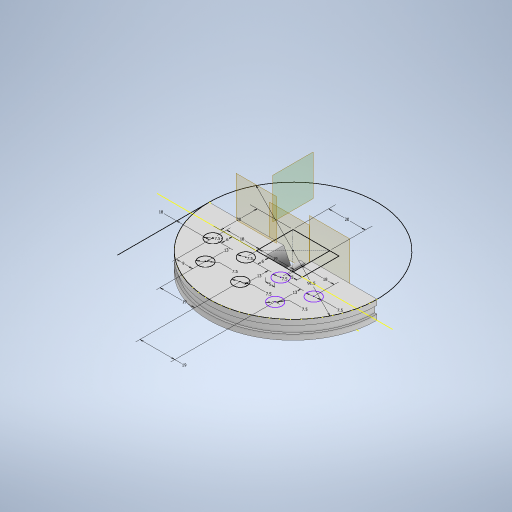
# Autodesk Inventor part: new탄두윗판구멍1_2
Saved by Autodesk Inventor 2023 (Build 270158000, 158)
## iProperties
Created: 2023-10-30
Part Number: new탄두윗판구멍1_2
Material: 일반
Document SubType Name: Modeling
Designer: rlatk
Density: 1 g/cm^3
Appearance: 기본값
Author: rlatk
Autodesk Inventor part; units mm, degrees
ref_plane "YZ Plane" through (0, 0, 0) normal (1, 0, 0) x (0, 1, 0)
ref_plane "XZ Plane" through (0, 0, 0) normal (0, 1, 0) x (-1, 0, 0)
ref_plane "XY Plane" through (0, 0, 0) normal (0, 0, 1) x (1, 0, 0)
sketch "스케치1" plane through (0, 0, 0) normal (0, 1, 0) x (-1, 0, 0)
  line L0 (-10, 10) -> (10, 10)
  line L1 (10, 10) -> (10, -10)
  line L2 (10, -10) -> (-10, -10)
  line L3 (-10, -10) -> (-10, 10)
  line L4 (-10, 10) -> (10, -10) construction
  line L5 (10, 10) -> (-10, -10) construction
  line L6 (-10, -10) -> (-15, -10)
  line L7 (-15, -10) -> (-15, 10)
  line L8 (-15, 10) -> (-10, 10)
  line L9 (-10, 10) -> (-10, -10)
  circle A0 centre (0, 0) radius 45.75
  dimension "d0" = 20
  dimension "d1" = 20
  dimension "d2" = 5
  dimension "d17" = 91.5
  constraints: 20 end point, 4 parallel, 2 horizontal, 2 midpoint, 2 perpendicular, 1 centre point, 1 coincident
  measures "d0" distance of L1.end L2.end
  measures "d1" distance of L0.end L1.end
  measures "d2" distance of L7.end L8.end
  measures "d17" diameter of A0
ref_plane "작업 평면2" through (-10, 20, -10) normal (-1, 0, 0) x (0, 0, 1)
sketch "스케치2" plane through (-10, 20, -10) normal (-1, 0, 0) x (0, 0, 1)
  line L0 (20, -100) -> (20, 0) projected
  line L1 (0, 0) -> (20, 0) projected
  line L2 (0, 0) -> (0, -100) projected
  line L3 (20, -100) -> (0, -100) projected
  circle A0 centre (10, -91) radius 4.5
  point P0 (10, -20)
  dimension "d7" = 9
  dimension "d8" = 9
  constraints: 1 centre point
  measures "d7" diameter of A0
  measures "d8" distance from line of L3 A0.centre
ref_plane "작업 평면1" through (-10, 20, 10) normal (0, 0, 1) x (1, 0, 0)
sketch "스케치3" plane through (-10, 20, 10) normal (0, 0, 1) x (1, 0, 0)
  line L0 (20, -20) -> (25, -20) projected
  line L1 (25, -20) -> (25, 0) projected
  line L2 (0, 0) -> (25, 0) projected
  line L3 (0, -100) -> (0, 0) projected
  line L4 (20, -100) -> (0, -100) projected
  line L5 (20, -20) -> (20, -100) projected
  line L6 (25, -20) -> (25, 0) projected
  line L7 (25, 0) -> (0, 0) projected
  arc A0 (25, -20) -> (20, 0) centre (-10.6945, -18.2986) ccw
  line L8 (20, 0) -> (25, 0)
  line L9 (25, 0) -> (25, -20)
  point P0 (10, -20)
  point P1 (20, 0)
  point P2 (25, -16.5972)
  constraints: 4 end point, 2 collinear, 2 point on circle, 1 centre point, 1 point on line
extrude "돌출4" [suppressed]
extrude "돌출5" [suppressed]
extrude "돌출6" add sketch "스케치1" against normal blind 10
ref_plane "작업 평면3" through (10, 0, -10) normal (0, 0, 1) x (1, 0, 0)
sketch "스케치4" plane through (10, 0, -10) normal (0, 0, 1) x (1, 0, 0)
  line L0 (0, -5) -> (-10, -5) projected
  line L1 (-10, -5) -> (-10, -80) projected
  line L2 (0, -80) -> (-10, -80) projected
  line L3 (0, -5) -> (0, -80) projected
  line L4 (-10, 0) -> (0, 0) projected
  line L5 (0, 0) -> (5, 0) projected
  line L6 (5, 0) -> (5, 3.4028) projected
  arc A0 (5, 3.4028) -> (0, 20) centre (-30.6945, 1.7014) ccw projected
  line L7 (-10, 20) -> (0, 20) projected
  line L8 (-10, 20) -> (-10, 0) projected
  line L9 (0, -5) -> (5, -5)
  line L10 (5, -5) -> (5, 0)
  line L11 (5, 0) -> (0, 0)
  line L12 (0, 0) -> (0, -5)
  line L13 (-55.75, -5) -> (35.75, -5) projected
  line L14 (-10, 0) -> (-15, 0)
  line L15 (-15, 0) -> (-15, -5)
  line L16 (-15, -5) -> (-10, -5)
  line L17 (-10, -5) -> (-10, 0)
  line L18 (-15, 0) -> (-10, -5)
  line L19 (0, 0) -> (5, -5)
  dimension "d20" = 5
  constraints: 20 end point, 4 parallel, 2 horizontal, 2 perpendicular, 1 point on line
  measures "d20" distance of L16.end L15.end
sketch "스케치5" plane through (0, 0, 0) normal (0, 1, 0) x (1, 0, 0)
  circle A0 centre (0, 0) radius 45.75 projected
  line L0 (15, -10) -> (-10, -10) projected
  line L1 (-10, 10) -> (15, 10) projected
  line L2 (-12.2866, 10.5) -> (15, 10.5)
  line L3 (15, 10.5) -> (15, -10.5)
  line L4 (15, -10.5) -> (-12.2866, -10.5)
  line L5 (-12.2866, -10.5) -> (-12.2866, 10.5)
  line L6 (15, 10) -> (15, -10) projected
  line L7 (-10, -10) -> (-10, 10) projected
  dimension "d22" = 0.5
  constraints: 8 end point, 2 parallel, 1 horizontal, 1 perpendicular
  measures "d22" distance between parallel lines of L1 L2
extrude "돌출7" [suppressed]
sketch "스케치6" plane through (-12.2866, 0, -10.5) normal (0, 0, 1) x (1, 0, 0)
  line L0 (7.2866, 0) -> (12.2866, -5) projected
  line L1 (7.2866, 0) -> (7.2866, -5) projected
  line L2 (7.2866, -5) -> (12.2866, -5) projected
  line L3 (22.2866, 0) -> (27.2866, -5) projected
  line L4 (22.2866, 0) -> (22.2866, -5) projected
  line L5 (22.2866, -5) -> (27.2866, -5) projected
  point P0 (12.2866, 0)
extrude "돌출8" [suppressed]
extrude "돌출9" add sketch "스케치4" along normal blind 20.5 and the other way blind 0.5 contours L19 L5 L10
ref_plane "작업 평면4" through (-12.2866, -5, -10.5) normal (0, 0, 1) x (1, 0, 0)
sketch "스케치7" plane through (-12.2866, -5, -10.5) normal (0, 0, 1) x (1, 0, 0)
  line L0 (7.2866, 0) -> (7.2866, 5) projected
  line L1 (0, 5) -> (7.2866, 5) projected
  line L2 (0, 5) -> (0, 0) projected
  line L3 (7.2866, 0) -> (0, 0) projected
  line L4 (0, 5) -> (7.2866, 5)
  line L5 (7.2866, 5) -> (7.2866, 0)
  line L6 (7.2866, 0) -> (0, 0)
  line L7 (0, 0) -> (0, 5)
  point P0 (12.2866, 5)
  constraints: 8 end point, 2 parallel, 1 horizontal, 1 perpendicular
extrude "돌출10" add sketch "스케치7" along normal blind 21
sketch "스케치8" plane through (-5, 0, -10) normal (0, 0, 1) x (1, 0, 0)
  line L0 (0, 0) -> (0, -5) projected
  line L1 (20, -10) -> (-5, -10) projected
  line L2 (20, -5) -> (15, 0) projected
  line L3 (0, 0) -> (15, 0) projected
  line L4 (0, 0) -> (5, 0)
  line L5 (5, 0) -> (5, -10)
  line L6 (5, -10) -> (0, -10)
  line L7 (0, -10) -> (0, 0)
  line L8 (0, 0) -> (5, -10)
  line L9 (0, -5) -> (-5, -5) projected
  line L10 (-5, -5) -> (-5, -10) projected
  line L11 (20, -5) -> (20, -10) projected
  dimension "d33" = 5
  constraints: 10 end point, 2 parallel, 1 horizontal, 1 perpendicular, 1 point on line
  measures "d33" distance of L5.end L6.end
extrude "돌출11" add sketch "스케치8" along normal blind 21
sketch "스케치9" plane through (0, 0, 0) normal (0, 1, 0) x (1, 0, 0)
  line L0 (10, -10) -> (-10, -10) projected
  line L1 (10, 10) -> (10, -10) projected
  line L2 (64.05, 10) -> (-64.05, 10) projected
  line L3 (-10, -64.05) -> (-10, 64.05) projected
  line L4 (-10, -10) -> (-10, 10) projected
  line L5 (-10, 10) -> (10, 10) projected
  line L6 (10, -10) -> (0, -10)
  line L7 (0, -10) -> (0, 10)
  line L8 (0, 10) -> (10, 10)
  line L9 (10, 10) -> (10, -10)
  point P0 (0, 0)
  constraints: 8 end point, 2 parallel, 1 horizontal, 1 midpoint, 1 perpendicular
extrude "돌출12" cut sketch "스케치9" against normal blind 10 contours L0 L7 L2 L1
sketch "스케치10" plane through (10, 0, 10) normal (0, 0, -1) x (-1, 0, 0)
  line L0 (-5, 0) -> (0, 0) projected
  line L1 (0, 0) -> (0, -10) projected
  line L2 (-35.75, -10) -> (55.75, -10) projected
  line L3 (0, 0) -> (-5, 0)
  line L4 (-5, 0) -> (-5, -10)
  line L5 (-5, -10) -> (0, -10)
  line L6 (0, -10) -> (0, 0)
  line L7 (0, 0) -> (-5, -10)
  line L8 (10, 0) -> (15, 0)
  line L9 (15, 0) -> (15, -10)
  line L10 (15, -10) -> (10, -10)
  line L11 (10, -10) -> (10, 0)
  line L12 (15, 0) -> (10, -10)
  dimension "d38" = 5
  constraints: 20 end point, 4 parallel, 2 horizontal, 2 perpendicular, 2 point on line
  measures "d38" distance of L9.end L10.end
extrude "돌출13" cut sketch "스케치10" along normal blind 20 contours L11 L8 L12
extrude "돌출14" cut sketch "스케치10" along normal blind 20 contours L1 L2 L7
sketch "스케치11" plane through (10, 0, 10) normal (0, 0, -1) x (-1, 0, 0)
  line L0 (-35.75, -10) -> (55.75, -10) projected
  line L1 (55.75, 0) -> (-35.75, 0) projected
  line L2 (0, 0) -> (0, -10) projected
  line L3 (10, -10) -> (10, 0) projected
  line L4 (0, 0) -> (10, 0)
  line L5 (10, 0) -> (10, -10)
  line L6 (10, -10) -> (0, -10)
  line L7 (0, -10) -> (0, 0)
  circle A0 centre (5, -5) radius 2.5
  dimension "d43" = 5
  constraints: 8 end point, 2 parallel, 1 centre point, 1 coincident, 1 horizontal, 1 perpendicular
  measures "d43" diameter of A0
extrude "돌출15" add sketch "스케치11" along normal blind 20 contours A0
sketch "스케치12" plane through (0, 0, 0) normal (0, 0, 1) x (1, 0, 0)
  line L0 (-45.75, -10) -> (45.75, -10) projected
  line L1 (45.75, 0) -> (-45.75, 0) projected
  line L2 (-45.75, -10) -> (45.75, -10) projected
  line L3 (-45.75, 0) -> (45.75, 0)
  line L4 (45.75, 0) -> (45.75, -10)
  line L5 (45.75, -10) -> (-45.75, -10)
  line L6 (-45.75, -10) -> (-45.75, 0)
  point P0 (0, 0)
  constraints: 8 end point, 2 parallel, 1 horizontal, 1 perpendicular
extrude "돌출16" cut sketch "스케치12" against normal blind 50
sketch "스케치13" plane through (0, 0, 0) normal (0, 0, -1) x (-1, 0, 0)
  line L0 (13.75, -2.95) -> (38.85, -2.95)
  line L1 (38.85, -2.95) -> (38.85, -7.05)
  line L2 (38.85, -7.05) -> (13.75, -7.05)
  line L3 (13.75, -7.05) -> (13.75, -2.95)
  line L4 (-41.1, -2.95) -> (-21, -2.95)
  line L5 (-21, -2.95) -> (-21, -7.05)
  line L6 (-21, -7.05) -> (-41.1, -7.05)
  line L7 (-41.1, -7.05) -> (-41.1, -2.95)
  line L8 (45.75, 0) -> (45.75, -10) projected
  line L9 (-45.75, 0) -> (-45.75, -10) projected
  line L10 (-45.75, 0) -> (-10, 0) projected
  line L11 (5, 0) -> (45.75, 0) projected
  point P0 (0, 0)
  dimension "d48" = 25.1
  dimension "d49" = 4.1
  dimension "d50" = 20.1
  dimension "d51" = 4.1
  dimension "d52" = 6.9
  dimension "d53" = 4.65
  dimension "d54" = 2.95
  dimension "d55" = 2.95
  constraints: 16 end point, 4 parallel, 2 horizontal, 2 perpendicular
  measures "d48" distance of L1.end L2.end
  measures "d49" distance of L0.end L1.end
  measures "d50" distance of L5.end L6.end
  measures "d51" distance of L4.end L5.end
  measures "d52" distance between parallel lines of L1 L8
  measures "d53" distance between parallel lines of L9 L7
  measures "d54" distance between parallel lines of L4 L10
  measures "d55" distance between parallel lines of L0 L11
extrude "돌출17" cut sketch "스케치13" against normal blind 5
sketch "스케치14" plane through (0, 0, 0) normal (0, 0, -1) x (-1, 0, 0)
  line L0 (38.85, -2.95) -> (38.85, -7.05) projected
  line L1 (38.85, -7.05) -> (13.75, -7.05) projected
  line L2 (13.75, -7.05) -> (13.75, -2.95) projected
  line L3 (13.75, -2.95) -> (38.85, -2.95) projected
  line L4 (0, -10) -> (5, 0) projected
  line L5 (45.75, -10) -> (0, -10) projected
  line L6 (45.75, 0) -> (45.75, -10) projected
  line L7 (5, 0) -> (45.75, 0) projected
  line L8 (45.75, -2.95) -> (44.55, -2.95)
  line L9 (44.55, -2.95) -> (44.55, -7.05)
  line L10 (44.55, -7.05) -> (45.75, -7.05)
  line L11 (45.75, -7.05) -> (45.75, -2.95)
  line L12 (0, -12) -> (0, 2) projected
  point P0 (0, 0)
  dimension "d58" = 1.2
  constraints: 8 end point, 2 parallel, 1 horizontal, 1 perpendicular, 1 point on line
  measures "d58" distance of L10.end L9.end
revolve "회전1" cut sketch "스케치14" angle 360 about axis through (0, -10, 0) along (0, 1, 0) contours L10 L9 L8 L6
sketch "스케치15" plane through (0, 0, 0) normal (0, 1, 0) x (1, 0, 0)
  circle A0 centre (-27.75, -16) radius 3.75
  circle A1 centre (-9.75, -16) radius 3.75
  circle A2 centre (9.25, -16) radius 3.75
  circle A3 centre (27.25, -16) radius 3.75
  circle A4 centre (-18.75, -29) radius 3.75
  circle A5 centre (0.25, -29) radius 3.75
  circle A6 centre (19.25, -29) radius 3.75
  line L0 (-44.55, 0) -> (-45.75, 0) projected
  line L1 (-45.75, 0) -> (-45.75, -49.8385)
  arc A7 (-45.75, 0) -> (45.75, 0) centre (0, 0) ccw projected
  line L2 (64.05, -10) -> (-64.05, -10) projected
  dimension "d60" = 7.5
  dimension "d61" = 7.5
  dimension "d62" = 7.5
  dimension "d63" = 7.5
  dimension "d64" = 7.5
  dimension "d65" = 7.5
  dimension "d66" = 7.5
  dimension "d67" = 18
  dimension "d68" = 18
  dimension "d69" = 19
  dimension "d70" = 18
  dimension "d71" = 9
  dimension "d72" = 19
  dimension "d73" = 19
  dimension "d74" = 13
  dimension "d75" = 13
  dimension "d76" = 13
  dimension "d77" = 6
  dimension "d78" = 6
  constraints: 7 centre point, 2 end point, 1 tangent, 1 vertical
  measures "d60" diameter of A0
  measures "d61" diameter of A1
  measures "d62" diameter of A2
  measures "d63" diameter of A3
  measures "d64" diameter of A4
  measures "d65" diameter of A5
  measures "d66" diameter of A6
  measures "d67" distance from line of L1 A0.centre
  measures "d68" distance of A1.centre A0.centre
  measures "d69" distance of A2.centre A1.centre
  measures "d70" distance of A2.centre A3.centre
  measures "d71" horizontal distance of A0.centre A4.centre
  measures "d72" distance of A5.centre A4.centre
  measures "d73" distance of A5.centre A6.centre
  measures "d74" vertical distance of A4.centre A0.centre
  measures "d75" vertical distance of A5.centre A1.centre
  measures "d76" vertical distance of A6.centre A2.centre
  measures "d77" distance from line of A1.centre L2
  measures "d78" distance from line of A0.centre L2
sketch "스케치16" plane through (0, -10, 0) normal (0, -1, 0) x (1, 0, 0)
  circle A0 centre (27.25, 16) radius 3.75 projected
  circle A1 centre (9.25, 16) radius 3.75 projected
  circle A2 centre (-9.75, 16) radius 3.75 projected
  circle A3 centre (-27.75, 16) radius 3.75 projected
  circle A4 centre (-18.75, 29) radius 3.75 projected
  circle A5 centre (0.25, 29) radius 3.75 projected
  circle A6 centre (19.25, 29) radius 3.75 projected
  point P0 (0, 0)
extrude "돌출19" cut sketch "스케치16" against normal blind 5
